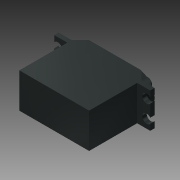
# Autodesk Inventor part: block
Saved by Autodesk Inventor 2015 (Build 190159000, 159)
## iProperties
Created: 2015-06-11
Part Number: block
Material: Generic
Document SubType Name: Modeling
Designer: david
Density: 1 g/cm^3
Appearance: Gunmetal - Polished
Mass: 28.6127 g
Surface Area: 64.4819 cm^2
Volume: 28.6127 cm^3
Author: david
Autodesk Inventor part; units mm, degrees
ref_plane "YZ Plane" through (0, 0, 0) normal (1, 0, 0) x (0, 1, 0)
ref_plane "XZ Plane" through (0, 0, 0) normal (0, 1, 0) x (-1, 0, 0)
ref_plane "XY Plane" through (0, 0, 0) normal (0, 0, 1) x (1, 0, 0)
sketch "Sketch1" plane through (0, 0, 0) normal (0, 1, 0) x (-1, 0, 0)
  line L0 (20, -10) -> (-20, -10)
  line L1 (-20, -10) -> (-20, 10)
  line L2 (-20, 10) -> (20, 10)
  line L3 (20, 10) -> (20, -10)
  line L4 (20, -10) -> (-20, 10) construction
  line L5 (-20, -10) -> (20, 10) construction
  point P0 (0, 0)
  dimension "d0" = 40
  dimension "d1" = 20
  constraints: 12 end point, 2 midpoint, 2 parallel, 1 horizontal, 1 perpendicular
  measures "d0" distance of L1.end L2.end
  measures "d1" distance of L0.end L1.end
extrude "Extrusion1" add sketch "Sketch1" along normal blind 30
sketch "Sketch2" plane through (20, 0, 10) normal (1, 0, 0) x (0, 0, -1)
  line L0 (0, 0) -> (0, 30) projected
  line L1 (20, 30) -> (0, 30)
  line L2 (0, 30) -> (0, 27.5)
  line L3 (0, 27.5) -> (20, 27.5)
  line L4 (20, 27.5) -> (20, 30)
  point P0 (10, 0)
  dimension "d4" = 2.5
  constraints: 8 end point, 2 parallel, 1 horizontal, 1 perpendicular, 1 point on line
  measures "d4" distance of L2.end L1.end
extrude "Extrusion2" add sketch "Sketch2" along normal blind 7.5
sketch "Sketch3" plane through (-20, 0, -10) normal (-1, 0, 0) x (0, 0, 1)
  line L0 (20, 0) -> (20, 30) projected
  line L1 (0, 30) -> (20, 30)
  line L2 (20, 30) -> (20, 27.5)
  line L3 (20, 27.5) -> (0, 27.5)
  line L4 (0, 27.5) -> (0, 30)
  point P0 (10, 0)
  dimension "d7" = 2.5
  constraints: 8 end point, 2 parallel, 1 horizontal, 1 perpendicular, 1 point on line
  measures "d7" distance of L1.end L2.end
extrude "Extrusion3" add sketch "Sketch3" along normal blind 7.5
sketch "Sketch4" plane through (0, 30, 0) normal (0, 1, 0) x (1, 0, 0)
  line L0 (20, 10) -> (-20, 10)
  line L1 (-20, 10) -> (-20, -10)
  line L2 (-20, -10) -> (20, -10)
  line L3 (20, -10) -> (20, 10)
  line L4 (20, 10) -> (-20, -10) construction
  line L5 (-20, 10) -> (20, -10) construction
  point P0 (0, 0)
  constraints: 12 end point, 2 midpoint, 2 parallel, 1 horizontal, 1 perpendicular
extrude "Extrusion4" add sketch "Sketch4" along normal blind 5
chamfer "Chamfer1" distance 5 angle 45 1 edges at (-20, 35, 0)
chamfer "Chamfer2" distance 5 angle 45 1 edges at (20, 35, 0)
sketch "Sketch5" plane through (0, 35, 0) normal (0, 1, 0) x (1, 0, 0)
  circle A0 centre (12.5, 0) radius 10
  line L0 (15, 10) -> (-15, 10) projected
  line L1 (27.5, 10) -> (27.5, -10) projected
  point P0 (0, 0)
  dimension "d18" = 15
  constraints: 1 centre point, 1 tangent
  measures "d18" distance from line of L1 A0.centre
extrude "Extrusion5" add sketch "Sketch5" against normal blind 5
sketch "Sketch6" plane through (0, 30, 0) normal (0, 1, 0) x (1, 0, 0)
  circle A0 centre (25.5, -5) radius 2.5
  line L0 (27.5, -10) -> (20, -10) projected
  line L1 (27.5, -10) -> (27.5, 10) projected
  circle A1 centre (25.5, 5) radius 2.5
  line L2 (20, 10) -> (27.5, 10) projected
  point P0 (0, 0)
  dimension "d21" = 5
  dimension "d22" = 5
  dimension "d23" = 2
  dimension "d24" = 5
  dimension "d25" = 5
  dimension "d26" = 2
  constraints: 2 centre point
  measures "d21" diameter of A0
  measures "d22" distance from line of L0 A0.centre
  measures "d23" distance from line of L1 A0.centre
  measures "d24" diameter of A1
  measures "d25" distance from line of L2 A1.centre
  measures "d26" distance from line of L1 A1.centre
extrude "Extrusion6" cut sketch "Sketch6" against normal blind 5
sketch "Sketch7" plane through (0, 30, 0) normal (0, 1, 0) x (1, 0, 0)
  circle A0 centre (-25.5, 5) radius 2.5
  circle A1 centre (-25.5, -5) radius 2.5
  line L0 (-27.5, -10) -> (-27.5, 10) projected
  line L1 (-20, -10) -> (-27.5, -10) projected
  line L2 (-27.5, 10) -> (-20, 10) projected
  point P0 (0, 0)
  dimension "d29" = 5
  dimension "d30" = 5
  dimension "d31" = 2
  dimension "d32" = 2
  dimension "d33" = 5
  dimension "d34" = 5
  constraints: 2 centre point
  measures "d29" diameter of A0
  measures "d30" diameter of A1
  measures "d31" distance from line of L0 A0.centre
  measures "d32" distance from line of L0 A1.centre
  measures "d33" distance from line of A1.centre L1
  measures "d34" distance from line of L2 A0.centre
extrude "Extrusion7" cut sketch "Sketch7" against normal blind 5
sketch "Sketch8" plane through (0, 35, 0) normal (0, 1, 0) x (1, 0, 0)
  circle A0 centre (12.5, 0) radius 5
  line L0 (27.5, 3.5) -> (27.5, -3.5) projected
  point P0 (0, 0)
  dimension "d37" = 10
  dimension "d38" = 15
  constraints: 1 centre point
  measures "d37" diameter of A0
  measures "d38" distance from line of A0.centre L0
extrude "Extrusion8" add sketch "Sketch8" along normal blind 2
sketch "Sketch9" plane through (12.5, 37, 0) normal (0, 1, 0) x (1, 0, 0)
  circle A0 centre (0, 0) radius 2.5
  point P0 (-12.5, 0)
  dimension "d41" = 5
  constraints: 1 centre point
  measures "d41" diameter of A0
extrude "Extrusion9" add sketch "Sketch9" along normal blind 4
sketch "Sketch10" plane through (-20, 0, -10) normal (-1, 0, 0) x (0, 0, 1)
  line L0 (13.25, 7.9352) -> (6.75, 7.9352)
  line L1 (6.75, 7.9352) -> (6.75, 4.9352)
  line L2 (6.75, 4.9352) -> (13.25, 4.9352)
  line L3 (13.25, 4.9352) -> (13.25, 7.9352)
  line L4 (13.25, 7.9352) -> (6.75, 4.9352) construction
  line L5 (6.75, 7.9352) -> (13.25, 4.9352) construction
  circle A0 centre (10, 6.4352) radius 1
  circle A1 centre (12.1728, 6.4352) radius 1
  circle A2 centre (7.7773, 6.4352) radius 1
  point P0 (10, 0)
  dimension "d44" = 6.5
  dimension "d45" = 3
  dimension "d46" = 2
  dimension "d47" = 2
  dimension "d48" = 2
  constraints: 12 end point, 3 centre point, 2 midpoint, 2 parallel, 1 coincident, 1 horizontal, 1 perpendicular
  measures "d44" distance of L2.end L1.end
  measures "d45" distance of L1.end L0.end
  measures "d46" diameter of A0
  measures "d47" diameter of A1
  measures "d48" diameter of A2
extrude "Extrusion10" add sketch "Sketch10" along normal blind 3
body "Solid1"
